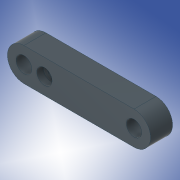
# Autodesk Inventor part: GA004
Saved by Autodesk Inventor 2017 (Build 210142000, 142)
## iProperties
Created: 2017-06-20
Part Number: GA004
Material: ABS Plastic
Document SubType Name: Modeling
Designer: zallen
Density: 1.06 g/cm^3
Appearance: CR Dark Blue
Author: zallen
Autodesk Inventor part; units mm, degrees
ref_plane "YZ Plane" through (0, 0, 0) normal (1, 0, 0) x (0, 1, 0)
ref_plane "XZ Plane" through (0, 0, 0) normal (0, 1, 0) x (-1, 0, 0)
ref_plane "XY Plane" through (0, 0, 0) normal (0, 0, 1) x (1, 0, 0)
sketch "Sketch1" plane through (0, 0, 0) normal (0, 0, 1) x (1, 0, 0)
  circle A0 centre (0, 0) radius 7.5 construction
  circle A1 centre (0, 0) radius 3.6
  arc A2 (0, 7.5) -> (0, -7.5) centre (0, 0) ccw
  line L0 (0, 7.5) -> (50, 7.5)
  line L1 (0, -7.5) -> (50, -7.5)
  circle A3 centre (50, 0) radius 7.5 construction
  arc A4 (50, -7.5) -> (50, 7.5) centre (50, 0) ccw
  circle A5 centre (50, 0) radius 3.5
  dimension "d0" = 15
  dimension "d1" = 7.2
  dimension "d2" = 50
  dimension "d3" = 7
  constraints: 8 point on circle, 6 centre point, 4 end point, 4 tangent, 3 coincident, 3 vertical alignment, 2 horizontal, 1 concentric
  measures "d0" diameter of A0
  measures "d1" diameter of A1
  measures "d2" distance of L0.start L0.end
  measures "d3" diameter of A5
extrude "Extrusion1" add sketch "Sketch1" along normal blind 10
sketch "Sketch2" plane through (0, 0, 10) normal (0, 0, 1) x (1, 0, 0)
  circle A0 centre (9.3, 0) radius 1.5
  point P0 (0, 0)
  dimension "d6" = 3
  dimension "d7" = 9.3
  constraints: 1 centre point, 1 horizontal alignment
  measures "d6" diameter of A0
  measures "d7" distance of A0.centre point (0, 0)
extrude "Extrusion2" cut sketch "Sketch2" against normal through all
sketch "Sketch3" plane through (0, 0, 10) normal (0, 0, 1) x (1, 0, 0)
  circle A0 centre (9.3, 0) radius 1.5 projected
  circle A1 centre (9.3, 0) radius 3.5
  point P0 (0, 0)
  dimension "d10" = 2
  constraints: 1 centre point
  measures "d10" radial gap between concentric circles of A0 A1
extrude "Extrusion3" cut sketch "Sketch3" against normal blind 3
body "Solid1"
